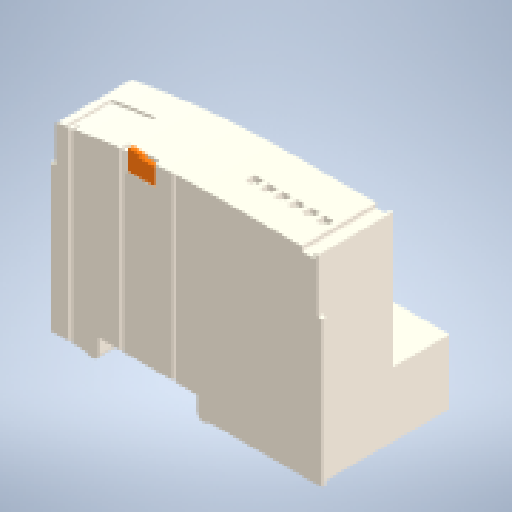
# Autodesk Inventor part: 750-354
Saved by Autodesk Inventor 2025.3 (Build 293356000, 356)
## iProperties
Category: PARTsolutions
Company: WAGO
Created: 2026-07-30
Part Number: 750-354
Material: Generic
Catalog Web Link: www.3dfindit.com
Description: 750-354-EtherCAT Fieldbus Coupler 100 mbit digital and analog signals
Vendor: WAGO
Document SubType Name: Modeling
Designer: psAdmin
Manufacturer: WAGO
Mass: 102.88 g
Surface Area: 329.615 cm^2
Volume: 209.864 cm^3
Density: 1 g/cm^3
Appearance: PSOLRGB-222-214-201
Categories: <MemberInstance><Categories><Category DisplayName="" Mnemonic="CABLEANDHARNESS" InternalName="e4a7e005-5e42-4d16-b293-125e7f0d0512"><Category DisplayName="" Mnemonic="CONNECTORS" InternalName="6f634eba-a678-4820-a31d-2c2d5ee6728e"><CategoryParameter DisplayName="" Mnemonic="REFDES" InternalName="c3740e8c-60ab-4d5d-8584-52b73222f2f0"/><Category DisplayName="" Mnemonic="DISCRETEWIRE" InternalName="9a3407de-09b2-4cdb-8c40-9708d5144a28"/></Category></Category></Categories><FamilyTemplate><FamilyTemplateParameters></FamilyTemplateParameters></FamilyTemplate><CategoryParameterMap><ParamToTemplateMap><ParamToTemplate CategoryParameter="//CategoryParameter[@InternalName='c3740e8c-60ab-4d5d-8584-52b73222f2f0']" ConstantValue=""/></ParamToTemplateMap></CategoryParameterMap></MemberInstance>
GlobalPropertyList: <PropertyList/>
PSOL_IDENT_0: {$CADENAS_DATA/23d-libs/wago/pg15/serie750/0750-0354_0999-0962.prj},157 {VTYP=3D},{NB=750-354},{LINA=
PSOL_IDENT_1: 750-354},{NN=750-354},{DATE=07.07.2026 11:01:27},{GEOMDATE=06.11.2024 07:19:12},{VERSION=},{LINEID=1
PSOL_IDENT_2: 180},{WBVAR=},{WBNUMERIC=}  {NB=750-354},{LINA=750-354},{KT=DUMMY},{BESTNR=750-354},{INFODE=Info DE}
PSOL_IDENT_3: ,{INFOEN=Info EN},{QUERSCHNITT1=0.08 - 1.5},{QUERSCHNITT2=28 - 14},{ABISOLIERLAENGE=5 - 6},{HOEHE=65
PSOL_IDENT_4: .00},{BREITE=50.00},{TIEFE=97.00},{FARBE=lichtgrau},{RGB=0.87,0.84,0.79,0},{GEWICHT=102.880},{ECLASS
PSOL_IDENT_5: 71=27-24-26-07},{LINKDE=http://www.wago.com/de/p/750-354},{LINKEN=http://www.wago.com/global/p/750-3
PSOL_IDENT_6: 54},{FILENAME=750-354}
NB: 750-354
NN: 750-354
NT: EtherCAT Fieldbus Coupler 100 mbit digital and analog signals
NBSYN: $BESTNR.
LINA: 750-354
CATALOG: WAGO
OFFICIAL_STANDARD_NUMBERS: NO
BESTNR: 750-354
INFODE: Info DE
INFOEN: Info EN
QUERSCHNITT1: 0.08 - 1.5
QUERSCHNITT2: 28 - 14
ABISOLIERLAENGE: 5 - 6
HOEHE: 65
BREITE: 50
TIEFE: 97
FARBE: lichtgrau
GEWICHT: 102.88
ECLASS71: 27-24-26-07
SUPPLIER: WAGO
ARTICLENO: 750-354
BOMINFO: 750-354
CREATOR: CADENAS GmbH
Title: 750-354
Author: Cadenas PARTsolutions
Comments: EtherCAT Fieldbus Coupler 100 mbit digital and analog signals
Autodesk Inventor part; units mm, degrees
ref_plane "YZ Plane" through (0, 0, 0) normal (1, 0, 0) x (0, 1, 0)
ref_plane "XZ Plane" through (0, 0, 0) normal (0, 1, 0) x (-1, 0, 0)
ref_plane "XY Plane" through (0, 0, 0) normal (0, 0, 1) x (1, 0, 0)
sketch "Skizze_13" plane through (0, 0, 2.5) normal (0, 0, 1) x (1, 0, 0)
  line L0 (-33, 23) -> (-33, -6.4)
  line L1 (-33, -6.4) -> (-22.2, -6.4)
  line L2 (-22.2, -6.4) -> (-20.582, -7.195)
  arc A0 (-20.582, -7.195) -> (-17.7, -5.4) centre (-19.7, -5.4) ccw
  line L3 (-17.7, -5.4) -> (-17.7, 0)
  line L4 (-17.7, 0) -> (17.7, 0)
  line L5 (17.7, 0) -> (17.7, -5.4)
  arc A1 (17.7, -5.4) -> (20.582, -7.195) centre (19.7, -5.4) ccw
  line L6 (20.582, -7.195) -> (22.2, -6.4)
  line L7 (22.2, -6.4) -> (60.6, -6.4)
  line L8 (60.6, -6.4) -> (60.6, 16.6)
  line L9 (60.6, 16.6) -> (21.6, 16.6)
  line L10 (21.6, 16.6) -> (21.6, 18.8)
  line L11 (21.6, 18.8) -> (9.2, 18.8)
  line L12 (9.2, 18.8) -> (9.2, 23)
  line L13 (9.2, 23) -> (-33, 23)
  constraints: 28 end point, 4 point on circle, 2 centre point
extrude "Extrusion1" add sketch "Skizze_13" along normal blind 20.3
sketch "Skizze_62" plane through (0, 0, 2.5) normal (0, 0, 1) x (1, 0, 0)
  arc A0 (8.3247, 3.5958) -> (8.9792, 2.5734) centre (9.3213, 3.5131) ccw
  line L0 (8.9792, 2.5734) -> (15.0029, 0.3809)
  arc A1 (15.0029, 0.3809) -> (16.029, 0.2) centre (16.029, 3.2) ccw
  line L1 (16.029, 0.2) -> (17.75, 0.2)
  line L2 (17.75, 0.2) -> (17.75, -1.1)
  line L3 (17.75, -1.1) -> (16.3, -1.4885)
  arc A2 (16.3, -1.4885) -> (16.8452, -3.1361) centre (30.8122, 2.4) ccw
  arc A3 (16.8452, -3.1361) -> (18.1418, -3.6978) centre (17.7749, -2.7676) ccw
  arc A4 (18.1418, -3.6978) -> (21.0155, 7.6281) centre (15.5, 3) ccw
  arc A5 (21.0155, 7.6281) -> (20.0963, 6.8567) centre (20.5559, 7.2424) ccw
  arc A6 (19.3302, 6.2139) -> (20.0963, 6.8567) centre (19.7132, 6.5353) ccw
  arc A7 (19.3302, 6.2139) -> (10.576, 3.8682) centre (15.5, 3) ccw
  arc A8 (9.5912, 4.0419) -> (10.576, 3.8682) centre (10.0836, 3.9551) ccw
  arc A9 (9.5912, 4.0419) -> (8.4094, 4.2503) centre (9.0003, 4.1461) ccw
  arc A10 (8.4094, 4.2503) -> (8.3247, 3.5958) centre (15.5, 3) ccw
  constraints: 22 point on circle, 11 centre point, 8 end point
extrude "Extrusion2" add sketch "Skizze_62" against normal blind 2.5
sketch "Skizze_63" plane through (0, 0, 22.8) normal (0, 0, 1) x (1, 0, 0)
  line L0 (-33, 58.4) -> (-33, -6.4)
  line L1 (-33, -6.4) -> (-22.2, -6.4)
  line L2 (-22.2, -6.4) -> (-20.582, -7.195)
  arc A0 (-20.582, -7.195) -> (-17.7, -5.4) centre (-19.7, -5.4) ccw
  line L3 (-17.7, -5.4) -> (-17.7, 0)
  line L4 (-17.7, 0) -> (17.7, 0)
  line L5 (17.7, 0) -> (17.7, -5.4)
  arc A1 (17.7, -5.4) -> (20.582, -7.195) centre (19.7, -5.4) ccw
  line L6 (20.582, -7.195) -> (22.2, -6.4)
  line L7 (22.2, -6.4) -> (60.6, -6.4)
  line L8 (60.6, -6.4) -> (60.6, 64.5)
  line L9 (60.6, 64.5) -> (24.6, 64.5)
  arc A2 (24.6, 64.5) -> (-32.5019, 58.8981) centre (25.2054, -235.4994) ccw
  line L10 (-32.5019, 58.8981) -> (-33, 58.4)
  constraints: 22 end point, 6 point on circle, 3 centre point
extrude "Extrusion3" add sketch "Skizze_63" along normal blind 26.7
sketch "Skizze_1" plane through (0, 0, 0) normal (1, 0, 0) x (0, 1, 0)
  line L0 (-8.4, 48) -> (-8.4, 4)
  line L1 (-8.4, 4) -> (-6.4, 4)
  line L2 (-6.4, 4) -> (-6.4, 48)
  line L3 (-6.4, 48) -> (-8.4, 48)
  constraints: 8 end point
extrude "Extrusion4" cut sketch "Skizze_1" along normal mid plane 50
sketch "Skizze_64" plane through (0, 64.5, 0) normal (0, 1, 0) x (1, 0, 0)
  line L0 (24.6, -36.1) -> (24.6, -39.3)
  line L1 (24.6, -39.3) -> (27.8, -39.3)
  line L2 (27.8, -39.3) -> (27.8, -36.1)
  line L3 (27.8, -36.1) -> (24.6, -36.1)
  constraints: 8 end point
extrude "Extrusion5" cut sketch "Skizze_64" against normal blind 2
pattern_linear "Rectangular Pattern1" count 6 spacing 5 along (1, 0, 0) of "Extrusion5"
sketch "Skizze_66" plane through (0, 0, 22.8) normal (0, 0, 1) x (1, 0, 0)
  arc A0 (54.8988, 63.8457) -> (54.59, 64.5) centre (54.59, 64.1) ccw
  line L0 (54.8988, 63.8457) -> (54.7718, 63.6915)
  arc A1 (54.7718, 63.6915) -> (54.8035, 63.0335) centre (55.15, 63.38) ccw
  line L1 (54.8035, 63.0335) -> (54.957, 62.88)
  line L2 (54.957, 62.88) -> (59.243, 62.88)
  line L3 (59.243, 62.88) -> (59.3965, 63.0335)
  arc A2 (59.3965, 63.0335) -> (59.4282, 63.6915) centre (59.05, 63.38) ccw
  line L4 (59.4282, 63.6915) -> (59.3012, 63.8457)
  arc A3 (59.61, 64.5) -> (59.3012, 63.8457) centre (59.61, 64.1) ccw
  line L5 (59.61, 64.5) -> (54.59, 64.5)
  constraints: 12 end point, 8 point on circle, 4 centre point
extrude "Extrusion6" cut sketch "Skizze_66" along normal blind 26.7
sketch "Skizze_71" plane through (0, 0, 49.1) normal (0, 0, 1) x (1, 0, 0)
  arc A0 (-13.3, 61.103) -> (-29.4, 58.5047) centre (26.4292, -236.2547) ccw
  line L0 (-13.3, 61.103) -> (-13.3, 62.103)
  arc A1 (-13.3, 62.103) -> (-29.4, 59.5047) centre (26.4292, -235.2547) ccw
  line L1 (-29.4, 59.5047) -> (-29.4, 58.5047)
  constraints: 4 end point, 4 point on circle, 2 centre point
extrude "Extrusion7" cut sketch "Skizze_71" against normal blind 15.85
sketch "Skizze_2" plane through (0, 18.8, 0) normal (0, 1, 0) x (1, 0, 0)
  line L0 (10.7, -17.9) -> (19.5, -17.9)
  line L1 (19.5, -17.9) -> (19.5, -5.1)
  line L2 (19.5, -5.1) -> (10.7, -5.1)
  line L3 (10.7, -5.1) -> (10.7, -17.9)
  constraints: 8 end point
extrude "Extrusion8" cut sketch "Skizze_2" against normal blind 2
sketch "Sketch_2" plane through (10.85, 0, 0) normal (1, 0, 0) x (0, 0, -1)
  line L0 (-17.8, 18.3) -> (-17.8, 7)
  arc A0 (-17.8, 7) -> (-17.6, 6.8) centre (-17.6, 7) ccw
  line L1 (-17.6, 6.8) -> (-4.6, 6.8)
  arc A1 (-4.6, 6.8) -> (-4.4, 7) centre (-4.6, 7) ccw
  line L2 (-4.4, 7) -> (-4.4, 16.8)
  line L3 (-4.4, 16.8) -> (-6.1, 18.8)
  line L4 (-6.1, 18.8) -> (-17.3, 18.8)
  arc A2 (-17.3, 18.8) -> (-17.8, 18.3) centre (-17.3, 18.3) ccw
  constraints: 10 end point, 6 point on circle, 3 centre point
extrude "Extrusion9" add sketch "Sketch_2" along normal blind 4.9
sketch "Sketch_3" plane through (15.75, 0, 0) normal (1, 0, 0) x (0, 0, -1)
  line L0 (-17.8, 18.3) -> (-17.8, 7)
  arc A0 (-17.8, 7) -> (-17.6, 6.8) centre (-17.6, 7) ccw
  line L1 (-17.6, 6.8) -> (-4.6, 6.8)
  arc A1 (-4.6, 6.8) -> (-4.4, 7) centre (-4.6, 7) ccw
  line L2 (-4.4, 7) -> (-4.4, 16.8)
  line L3 (-4.4, 16.8) -> (-6.1, 18.8)
  line L4 (-6.1, 18.8) -> (-17.3, 18.8)
  arc A2 (-17.3, 18.8) -> (-17.8, 18.3) centre (-17.3, 18.3) ccw
  constraints: 10 end point, 6 point on circle, 3 centre point
extrude "Extrusion10" add sketch "Sketch_3" along normal blind 3.5
sketch "Sketch_4" plane through (0, 18.8, 0) normal (0, 1, 0) x (1, 0, 0)
  line L0 (12.25, -12.05) -> (12.25, -14.95)
  line L1 (12.25, -14.95) -> (15.15, -14.95)
  line L2 (15.15, -14.95) -> (15.15, -12.05)
  line L3 (15.15, -12.05) -> (12.25, -12.05)
  constraints: 8 end point
extrude "Extrusion11" cut sketch "Sketch_4" against normal blind 1
sketch "Sketch_5" plane through (0, 18.8, 0) normal (0, 1, 0) x (1, 0, 0)
  line L0 (12.25, -6.65) -> (12.25, -10.75)
  line L1 (12.25, -10.75) -> (15.15, -10.75)
  line L2 (15.15, -10.75) -> (15.15, -6.65)
  line L3 (15.15, -6.65) -> (12.25, -6.65)
  constraints: 8 end point
extrude "Extrusion12" cut sketch "Sketch_5" against normal blind 1
sketch "Sketch_6" plane through (0, 18.8, 0) normal (0, 1, 0) x (1, 0, 0)
  line L0 (15.75, -12.05) -> (15.75, -14.95)
  line L1 (15.75, -14.95) -> (18.65, -14.95)
  line L2 (18.65, -14.95) -> (18.65, -12.05)
  line L3 (18.65, -12.05) -> (15.75, -12.05)
  constraints: 8 end point
extrude "Extrusion13" cut sketch "Sketch_6" against normal blind 1
sketch "Sketch_7" plane through (0, 18.8, 0) normal (0, 1, 0) x (1, 0, 0)
  line L0 (15.75, -6.65) -> (15.75, -10.75)
  line L1 (15.75, -10.75) -> (18.65, -10.75)
  line L2 (18.65, -10.75) -> (18.65, -6.65)
  line L3 (18.65, -6.65) -> (15.75, -6.65)
  constraints: 8 end point
extrude "Extrusion14" cut sketch "Sketch_7" against normal blind 1
sketch "Skizze_3" plane through (0, 23, 0) normal (0, 1, 0) x (1, 0, 0)
  line L0 (-28, -5.55) -> (-28, -22.75)
  line L1 (-28, -22.75) -> (-10.9, -22.75)
  line L2 (-10.9, -22.75) -> (-10.9, -5.55)
  line L3 (-10.9, -5.55) -> (-28, -5.55)
  constraints: 8 end point
extrude "Extrusion15" cut sketch "Skizze_3" against normal blind 11.3
sketch "Skizze_4" plane through (0, 23, 0) normal (0, 1, 0) x (1, 0, 0)
  line L0 (-9.1, -5.55) -> (-9.1, -22.75)
  line L1 (-9.1, -22.75) -> (8, -22.75)
  line L2 (8, -22.75) -> (8, -5.55)
  line L3 (8, -5.55) -> (-9.1, -5.55)
  constraints: 8 end point
extrude "Extrusion16" cut sketch "Skizze_4" against normal blind 11.3
sketch "Skizze_5" plane through (0, 23, 0) normal (0, 1, 0) x (1, 0, 0)
  line L0 (-27.5, -6.04) -> (-27.5, -22.74)
  line L1 (-27.5, -22.74) -> (-11.4, -22.74)
  line L2 (-11.4, -22.74) -> (-11.4, -6.04)
  line L3 (-11.4, -6.04) -> (-27.5, -6.04)
  line L4 (-25.35, -16.04) -> (-13.55, -16.04)
  line L5 (-13.55, -16.04) -> (-13.55, -9.04)
  line L6 (-13.55, -9.04) -> (-15.7, -9.04)
  line L7 (-15.7, -9.04) -> (-15.7, -7.54)
  line L8 (-15.7, -7.54) -> (-17.2, -7.54)
  line L9 (-17.2, -7.54) -> (-17.2, -6.29)
  line L10 (-17.2, -6.29) -> (-21.7, -6.29)
  line L11 (-21.7, -6.29) -> (-21.7, -7.54)
  line L12 (-21.7, -7.54) -> (-23.2, -7.54)
  line L13 (-23.2, -7.54) -> (-23.2, -9.04)
  line L14 (-23.2, -9.04) -> (-25.35, -9.04)
  line L15 (-25.35, -9.04) -> (-25.35, -16.04)
  constraints: 32 end point
extrude "Extrusion17" add sketch "Skizze_5" against normal blind 11.3
sketch "Skizze_6" plane through (0, 23, 0) normal (0, 1, 0) x (1, 0, 0)
  line L0 (-8.6, -6.04) -> (-8.6, -22.74)
  line L1 (-8.6, -22.74) -> (7.5, -22.74)
  line L2 (7.5, -22.74) -> (7.5, -6.04)
  line L3 (7.5, -6.04) -> (-8.6, -6.04)
  line L4 (-6.45, -16.04) -> (5.35, -16.04)
  line L5 (5.35, -16.04) -> (5.35, -9.04)
  line L6 (5.35, -9.04) -> (3.2, -9.04)
  line L7 (3.2, -9.04) -> (3.2, -7.54)
  line L8 (3.2, -7.54) -> (1.7, -7.54)
  line L9 (1.7, -7.54) -> (1.7, -6.29)
  line L10 (1.7, -6.29) -> (-2.8, -6.29)
  line L11 (-2.8, -6.29) -> (-2.8, -7.54)
  line L12 (-2.8, -7.54) -> (-4.3, -7.54)
  line L13 (-4.3, -7.54) -> (-4.3, -9.04)
  line L14 (-4.3, -9.04) -> (-6.45, -9.04)
  line L15 (-6.45, -9.04) -> (-6.45, -16.04)
  constraints: 32 end point
extrude "Extrusion18" add sketch "Skizze_6" against normal blind 11.3
sketch "Skizze_74" plane through (0, 0, 49.5) normal (0, 0, 1) x (1, 0, 0)
  line L0 (-7.4, 56.5) -> (2.6, 56.5)
  line L1 (2.6, 56.5) -> (2.6, 64.5)
  line L2 (2.6, 64.5) -> (-7.4, 64.5)
  line L3 (-7.4, 64.5) -> (-7.4, 56.5)
  constraints: 8 end point
extrude "Extrusion19" cut sketch "Skizze_74" against normal blind 1.9
sketch "Skizze_75" plane through (0, 0, 48.55) normal (0, 0, 1) x (1, 0, 0)
  line L0 (-7.1, 56.5) -> (2.3, 56.5)
  line L1 (2.3, 56.5) -> (2.3, 62)
  arc A0 (2.3, 62) -> (1.8, 62.5) centre (1.8, 62) ccw
  line L2 (1.8, 62.5) -> (-3.2, 62.5)
  arc A1 (-3.2305, 63.0984) -> (-3.2, 62.5) centre (-3.2, 62.8) ccw
  line L3 (-3.2305, 63.0984) -> (-2.2246, 63.2013)
  arc A2 (-2.2246, 63.2013) -> (-2.25, 63.7) centre (-2.25, 63.45) ccw
  line L4 (-2.25, 63.7) -> (-7.1, 63.7)
  line L5 (-7.1, 63.7) -> (-7.1, 56.5)
  constraints: 12 end point, 6 point on circle, 3 centre point
extrude "Extrusion20" add sketch "Skizze_75" along normal mid plane 1.6
sketch "Skizze_76" plane through (0, -6.4, 0) normal (0, 1, 0) x (1, 0, 0)
  line L0 (59.2, -48) -> (59.2, -49.5)
  line L1 (59.2, -49.5) -> (62.2, -49.5)
  line L2 (62.2, -49.5) -> (62.2, -48)
  line L3 (62.2, -48) -> (59.2, -48)
  constraints: 8 end point
extrude "Extrusion21" add sketch "Skizze_76" along normal blind 52
sketch "Skizze_77" plane through (0, -6.4, 0) normal (0, 1, 0) x (1, 0, 0)
  line L0 (-34.6, -48) -> (-34.6, -49.5)
  line L1 (-34.6, -49.5) -> (-31.6, -49.5)
  line L2 (-31.6, -49.5) -> (-31.6, -48)
  line L3 (-31.6, -48) -> (-34.6, -48)
  constraints: 8 end point
extrude "Extrusion22" add sketch "Skizze_77" along normal blind 52
sketch "Sketch_1" plane through (0, -10, 0) normal (0, 1, 0) x (1, 0, 0)
  line L0 (-28.1, -50.5) -> (9.7, -50.5)
  line L1 (9.7, -50.5) -> (9.7, -46.9)
  line L2 (9.7, -46.9) -> (8.7, -46.9)
  line L3 (8.7, -46.9) -> (8.7, -49.5)
  line L4 (8.7, -49.5) -> (-8.7, -49.5)
  line L5 (-8.7, -49.5) -> (-8.7, -46.9)
  line L6 (-8.7, -46.9) -> (-9.7, -46.9)
  line L7 (-9.7, -46.9) -> (-9.7, -49.5)
  line L8 (-9.7, -49.5) -> (-27.1, -49.5)
  line L9 (-27.1, -49.5) -> (-27.1, -46.9)
  line L10 (-27.1, -46.9) -> (-28.1, -46.9)
  line L11 (-28.1, -46.9) -> (-28.1, -50.5)
  constraints: 24 end point
extrude "Extrusion23" cut sketch "Sketch_1" along normal blind 74
body "Solid1"
